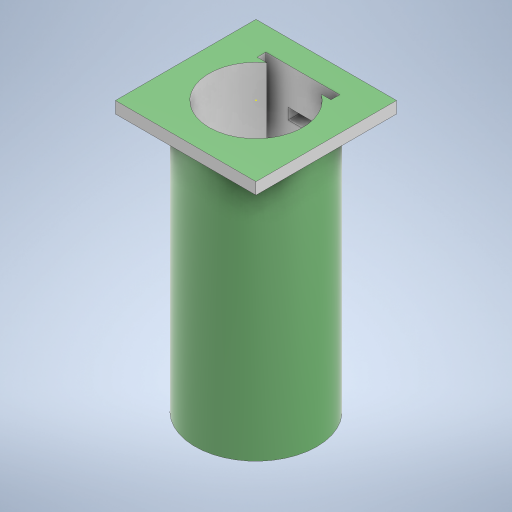
# Autodesk Inventor part: WaterCollector
Saved by Autodesk Inventor 2023 (Build 270158000, 158)
## iProperties
Created: 2023-09-26
Part Number: WaterCollector
Material: Generic
Document SubType Name: Modeling
Designer: Gage
Density: 1 g/cm^3
Appearance: Default
Author: Gage
## iProperties of the stored document WaterCollector_3DPrint.ipt
Created: 2023-10-03
Part Number: WaterCollector_3DPrint
Material: Generic
Document SubType Name: Modeling
Designer: Gage
Density: 1 g/cm^3
Appearance: Default
Author: Gage
Autodesk Inventor part; units mm, degrees
ref_plane "YZ Plane" through (0, 0, 0) normal (1, 0, 0) x (0, 1, 0)
ref_plane "XZ Plane" through (0, 0, 0) normal (0, 1, 0) x (-1, 0, 0)
ref_plane "XY Plane" through (0, 0, 0) normal (0, 0, 1) x (1, 0, 0)
sketch "Sketch1" plane through (0, 0, 0) normal (0, 1, 0) x (-1, 0, 0)
  line L0 (31.75, -31.75) -> (-31.75, -31.75)
  line L1 (-31.75, -31.75) -> (-31.75, 31.75)
  line L2 (-31.75, 31.75) -> (31.75, 31.75)
  line L3 (31.75, 31.75) -> (31.75, -31.75)
  point P0 (0, 0)
  point P1 (-31.75, 0)
  point P2 (0, -31.75)
  dimension "d0" = 63.5
  dimension "d1" = 63.5
  constraints: 8 end point, 2 midpoint, 2 parallel, 1 horizontal, 1 horizontal alignment, 1 perpendicular, 1 vertical alignment
  measures "d0" distance of L1.end L2.end
  measures "d1" distance of L0.end L1.end
extrude "Extrusion1" add sketch "Sketch1" along normal blind 69.85
sketch "Sketch2" plane through (0, 69.85, 0) normal (0, 1, 0) x (1, 0, 0)
  circle A0 centre (0, 0) radius 12.7
  line L0 (-10, 12.7) -> (10, 12.7)
  line L1 (10, 12.7) -> (10, 10.3187)
  line L2 (10, 10.3187) -> (-10, 10.3187)
  line L3 (-10, 10.3187) -> (-10, 12.7)
  point P0 (-12.7, 0)
  point P1 (12.7, 0)
  point P2 (0, 12.7)
  point P3 (-7.4036, 10.3187)
  point P4 (0, 7.5)
  point P5 (7.4036, 10.3187)
  dimension "d4" = 25.4
  dimension "d7" = 20
  dimension "d8" = 2.3813
  constraints: 8 end point, 3 point on circle, 2 parallel, 1 centre point, 1 coincident, 1 horizontal, 1 midpoint, 1 perpendicular, 1 vertical alignment
  measures "d4" diameter of A0
  measures "d7" distance of L1.end L2.end
  measures "d8" distance between parallel lines of L2 L0
extrude "Extrusion2" cut sketch "Sketch2" against normal through all
sketch "Sketch4" plane through (0, 69.85, 0) normal (0, 1, 0) x (1, 0, 0)
  circle A0 centre (0, 0) radius 16.51
  line L0 (-23.2494, 25.4) -> (-10.5494, 25.4)
  line L1 (-10.5494, 25.4) -> (-10.5494, 12.7)
  line L2 (-10.5494, 12.7) -> (-23.2494, 12.7)
  line L3 (-23.2494, 12.7) -> (-23.2494, 25.4)
  line L4 (-31.75, 31.75) -> (-31.75, -31.75) projected
  line L5 (-31.75, 0) -> (31.75, 0)
  line L6 (10.5494, 25.4) -> (23.2494, 25.4)
  line L7 (23.2494, 25.4) -> (23.2494, 12.7)
  line L8 (23.2494, 12.7) -> (10.5494, 12.7)
  line L9 (10.5494, 12.7) -> (10.5494, 25.4)
  line L10 (10.5494, -12.7) -> (23.2494, -12.7)
  line L11 (23.2494, -12.7) -> (23.2494, -25.4)
  line L12 (23.2494, -25.4) -> (10.5494, -25.4)
  line L13 (10.5494, -25.4) -> (10.5494, -12.7)
  line L14 (-23.2494, -12.7) -> (-10.5494, -12.7)
  line L15 (-10.5494, -12.7) -> (-10.5494, -25.4)
  line L16 (-10.5494, -25.4) -> (-23.2494, -25.4)
  line L17 (-23.2494, -25.4) -> (-23.2494, -12.7)
  line L18 (-23.2494, 25.4) -> (23.2494, 25.4)
  line L19 (23.2494, 25.4) -> (23.2494, -25.4)
  line L20 (23.2494, -25.4) -> (-23.2494, -25.4)
  line L21 (-23.2494, -25.4) -> (-23.2494, 25.4)
  line L22 (31.75, -31.75) -> (31.75, 31.75) projected
  line L23 (-31.75, 31.75) -> (31.75, 31.75)
  line L24 (31.75, 31.75) -> (31.75, -31.75)
  line L25 (31.75, -31.75) -> (-31.75, -31.75)
  line L26 (-31.75, -31.75) -> (-31.75, 31.75)
  dimension "d10" = 33.02
  dimension "d11" = 12.7
  dimension "d12" = 12.7
  dimension "d13" = 12.7
  dimension "d14" = 12.7
  dimension "d15" = 12.7
  dimension "d16" = 12.7
  dimension "d17" = 12.7
  dimension "d18" = 12.7
  dimension "d19" = 12.7
  dimension "d20" = 12.7
  dimension "d21" = 12.7
  dimension "d22" = 12.7
  constraints: 50 end point, 12 parallel, 7 horizontal, 6 perpendicular, 4 point on circle, 1 centre point, 1 coincident, 1 midpoint
  measures "d10" diameter of A0
  measures "d11" distance of L1.end L2.end
  measures "d12" distance of L0.end L1.end
  measures "d13" distance between parallel lines of L2 L5
  measures "d14" distance of L7.end L8.end
  measures "d15" distance of L6.end L7.end
  measures "d16" distance of L11.end L12.end
  measures "d17" distance of L10.end L11.end
  measures "d18" distance of L15.end L16.end
  measures "d19" distance of L14.end L15.end
  measures "d20" distance between parallel lines of L5 L8
  measures "d21" distance between parallel lines of L5 L10
  measures "d22" distance between parallel lines of L5 L14
sketch "Sketch5" plane through (0, 69.85, 0) normal (0, 1, 0) x (1, 0, 0)
  point P0 (0, 0)
extrude "Extrusion3" cut sketch "Sketch4" against normal blind 50.8 contours L19 L7 L6 L18 L0 L3 L21 L5 L4 L23 L22 | L5 L22 L25 L4 L21 L17 L16 L20 L12 L11 L19
sketch "Sketch6" plane through (0, 69.85, 0) normal (0, 1, 0) x (1, 0, 0)
  point P0 (0, 0)
sketch "Sketch7" plane through (0, 0, 0) normal (0, -1, 0) x (1, 0, 0)
  circle A0 centre (0, 0) radius 16.51
  line L0 (-23.2494, 25.4) -> (23.2494, 25.4) projected
  line L1 (23.2494, 25.4) -> (23.2494, -25.4) projected
  line L2 (-23.2494, 25.4) -> (23.2494, 25.4)
  line L3 (23.2494, 25.4) -> (23.2494, -25.4)
  line L4 (23.2494, -25.4) -> (-23.2494, -25.4)
  line L5 (-23.2494, -25.4) -> (-23.2494, 25.4)
  dimension "d25" = 33.02
  constraints: 8 end point, 2 parallel, 1 centre point, 1 coincident, 1 horizontal, 1 perpendicular
  measures "d25" diameter of A0
extrude "Extrusion4" cut sketch "Sketch7" against normal blind 66.675
sketch "Sketch9" plane through (0, 69.85, 0) normal (0, 1, 0) x (1, 0, 0)
  line L0 (-19.05, 19.05) -> (19.05, 19.05)
  line L1 (19.05, 19.05) -> (19.05, -19.05)
  line L2 (19.05, -19.05) -> (-19.05, -19.05)
  line L3 (-19.05, -19.05) -> (-19.05, 19.05)
  line L4 (23.2494, -25.4) -> (23.2494, 25.4) projected
  line L5 (-23.2494, 25.4) -> (23.2494, 25.4)
  line L6 (23.2494, 25.4) -> (23.2494, -25.4)
  line L7 (23.2494, -25.4) -> (-23.2494, -25.4)
  line L8 (-23.2494, -25.4) -> (-23.2494, 25.4)
  line L9 (31.75, -31.75) -> (-31.75, -31.75) projected
  line L10 (-31.75, -31.75) -> (-31.75, 31.75) projected
  line L11 (31.75, -31.75) -> (-31.75, -31.75)
  line L12 (-31.75, -31.75) -> (-31.75, 31.75)
  line L13 (-31.75, 31.75) -> (31.75, 31.75)
  line L14 (31.75, 31.75) -> (31.75, -31.75)
  point P0 (0, 0)
  point P1 (0, 19.05)
  point P2 (19.05, 0)
  point P3 (23.2494, 25.4)
  dimension "d42" = 38.1
  dimension "d43" = 38.1
  constraints: 24 end point, 6 parallel, 3 horizontal, 3 perpendicular, 2 midpoint, 1 horizontal alignment, 1 vertical alignment
  measures "d42" distance of L1.end L2.end
  measures "d43" distance of L0.end L1.end
extrude "Extrusion6" cut sketch "Sketch9" against normal through all contours L7 L8 L5 L4 | L9 L10 L13 L14
sketch "Sketch21" plane through (0, 0, 0) normal (0, -1, 0) x (1, 0, 0)
  arc A0 (7.4036, -10.3187) -> (-7.4036, -10.3187) centre (0, 0) ccw projected
  circle A1 centre (0, 0) radius 16.51
  constraints: 1 centre point, 1 coincident
extrude "Extrusion15" add sketch "Sketch21" along normal blind 3.175
sketch "Sketch22" plane through (-10, 69.85, -12.7) normal (0, 0, 1) x (1, 0, 0)
  line L0 (20, -69.85) -> (0, -69.85) projected
  line L1 (6, -12.93) -> (14, -12.93)
  line L2 (14, -12.93) -> (14, -9.93)
  line L3 (14, -9.93) -> (6, -9.93)
  line L4 (6, -9.93) -> (6, -12.93)
  point P0 (10, -69.85)
  point P1 (10, -11.43)
  point P2 (14, -11.43)
  point P3 (10, -9.93)
  dimension "d87" = 58.42
  dimension "d88" = 8
  dimension "d89" = 3
  constraints: 8 end point, 2 midpoint, 2 parallel, 1 horizontal, 1 horizontal alignment, 1 perpendicular, 1 vertical alignment
  measures "d87" distance from line of L0 point (10, -11.43)
  measures "d88" distance of L3.end L2.end
  measures "d89" distance of L2.end L1.end
extrude "Extrusion16" cut sketch "Sketch22" against normal blind 6.35
body "Solid1"
